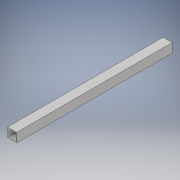
# Autodesk Inventor part: Vertical frame Extension 2
Saved by Autodesk Inventor 2017 (Build 210142000, 142)
## iProperties
Created: 2020-02-04
Part Number: Vertical frame Extension 2
Material: Generic
Document SubType Name: Modeling
Designer: S332848902
Density: 1 g/cm^3
Appearance: Default
Author: S332848902
Autodesk Inventor part; units mm, degrees
ref_plane "YZ Plane" through (0, 0, 0) normal (1, 0, 0) x (0, 1, 0)
ref_plane "XZ Plane" through (0, 0, 0) normal (0, 1, 0) x (-1, 0, 0)
ref_plane "XY Plane" through (0, 0, 0) normal (0, 0, 1) x (1, 0, 0)
sketch "Sketch1" plane through (0, 0, 0) normal (0, 0, 1) x (1, 0, 0)
  line L0 (12.7, -12.7) -> (-12.7, -12.7) projected
  line L1 (12.7, 12.7) -> (12.7, -12.7) projected
  line L2 (-12.7, 12.7) -> (12.7, 12.7) projected
  line L3 (-12.7, -12.7) -> (-12.7, 12.7) projected
  line L4 (10.16, 10.16) -> (10.16, -10.16) projected
  line L5 (10.16, -10.16) -> (-10.16, -10.16) projected
  line L6 (-10.16, -10.16) -> (-10.16, 10.16) projected
  line L7 (-10.16, 10.16) -> (10.16, 10.16) projected
  point P0 (0, 0)
extrude "Extrusion1" add sketch "Sketch1" along normal blind 431.8
body "Solid1"
